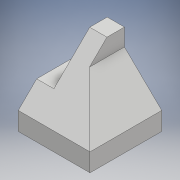
# Autodesk Inventor part: Part1
Saved by Autodesk Inventor 2018 (Build 220112000, 112)
## iProperties
Created: 2017-11-15
Part Number: Part1
Material: Generic
Document SubType Name: Modeling
Designer: kurti
Density: 1 g/cm^3
Appearance: Default
Author: kurti
Autodesk Inventor part; units mm, degrees
ref_plane "YZ Plane" through (0, 0, 0) normal (1, 0, 0) x (0, 1, 0)
ref_plane "XZ Plane" through (0, 0, 0) normal (0, 1, 0) x (-1, 0, 0)
ref_plane "XY Plane" through (0, 0, 0) normal (0, 0, 1) x (1, 0, 0)
sketch "Sketch1" plane through (0, 0, 0) normal (0, 0, 1) x (1, 0, 0)
  line L0 (-9.375, -9.375) -> (9.375, -9.375)
  line L1 (9.375, -9.375) -> (9.375, 9.375)
  line L2 (9.375, 9.375) -> (-9.375, 9.375)
  line L3 (-9.375, 9.375) -> (-9.375, -9.375)
  line L4 (-9.375, -9.375) -> (9.375, 9.375) construction
  line L5 (9.375, -9.375) -> (-9.375, 9.375) construction
  point P0 (0, 0)
  dimension "d0" = 18.75
  dimension "d1" = 18.75
  constraints: 12 end point, 2 midpoint, 2 parallel, 1 horizontal, 1 perpendicular
  measures "d0" distance of L1.end L2.end
  measures "d1" distance between parallel lines of L0 L2
extrude "Extrusion1" add sketch "Sketch1" along normal blind 18.75
sketch "Sketch2" plane through (9.375, -9.375, 0) normal (1, 0, 0) x (0, 0, -1)
  line L0 (0, 0) -> (-4.75, 0)
  line L1 (0, 0) -> (-18.75, 0) projected
  line L2 (-18.75, 18.6787) -> (-18.75, 14.1787)
  line L3 (-18.75, 0) -> (-18.75, 18.75) projected
  line L4 (-18.75, 14.1787) -> (-4.75, 0)
  line L5 (0, 0) -> (0, 18.6787)
  line L6 (0, 18.6787) -> (-18.75, 18.6787)
  line L7 (-18.75, 0) -> (-4.75, 0)
  line L8 (-18.75, 0) -> (-18.75, 14.1787)
  point P0 (0, 9.375)
  point P1 (-18.75, 18.75)
  dimension "d4" = 4.75
  dimension "d5" = 4.5
  dimension "d6" = 45.363
  dimension "d7" = 90.001
  constraints: 14 end point, 1 horizontal, 1 perpendicular, 1 point on line, 1 vertical, 2 other
  measures "d4" distance of L0.start L0.end
  measures "d5" distance of L2.start L2.end
  measures "d6" angle of L4 L1
  measures "d7" angle of L2 L1
extrude "Extrusion2" cut sketch "Sketch2" against normal blind 21 contours L1 L3 L4
sketch "Sketch3" plane through (-9.375, -9.375, 0) normal (0, -1, 0) x (1, 0, 0)
  line L0 (18.75, 18.75) -> (0, 18.75) projected
  line L1 (0, 18.75) -> (4.5, 18.75)
  line L2 (4.5, 18.75) -> (4.5, 9.5)
  line L3 (4.5, 9.5) -> (0, 9.5)
  line L4 (0, 9.5) -> (0, 18.75)
  line L5 (4.5, 18.75) -> (9, 18.75) construction
  line L6 (9, 18.75) -> (9, 14.25)
  line L7 (0, 0) -> (18.75, 0) construction
  line L8 (18.75, 0) -> (18.75, 4.75) construction
  line L9 (18.75, 0) -> (18.75, 18.75) construction
  line L10 (18.75, 4.75) -> (9, 14.25)
  line L11 (9, 18.75) -> (18.75, 18.75)
  line L12 (18.75, 4.75) -> (18.75, 18.75)
  point P0 (9.375, 0)
  dimension "d10" = 4.5
  dimension "d11" = 9.25
  dimension "d12" = 4.5
  dimension "d13" = 4.5
  dimension "d14" = 4.75
  constraints: 20 end point, 3 perpendicular, 2 parallel, 2 point on line, 1 collinear, 1 horizontal
  measures "d10" distance of L2.end L3.end
  measures "d11" distance between parallel lines of L3 L0
  measures "d12" distance of L1.end L5.end
  measures "d13" distance of L5.end L6.end
  measures "d14" distance of L7.end L8.end
extrude "Extrusion3" cut sketch "Sketch3" against normal blind 27.25
body "Solid1"
